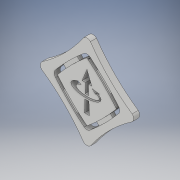
# Autodesk Inventor part: IEEE 3D
Saved by Autodesk Inventor 2018 (Build 220112000, 112)
## iProperties
Created: 2017-04-26
Part Number: IEEE 3D
Material: Generic
Document SubType Name: Modeling
Designer: Docente
Density: 1 g/cm^3
Appearance: Default
Author: Docente
Autodesk Inventor part; units mm, degrees
sketch "Sketch1" plane through (0, 0, 0) normal (0, 0, 1) x (1, 0, 0)
  line L0 (0, 0) -> (40, 0) construction
  line L1 (40, 0) -> (40, 40) construction
  line L2 (40, 40) -> (0, 40) construction
  line L3 (0, 40) -> (0, 0) construction
  line L4 (21.4142, 38.5858) -> (38.5858, 21.4142)
  line L5 (21.4142, 1.4142) -> (38.5858, 18.5858)
  line L6 (18.5858, 1.4142) -> (1.4142, 18.5858)
  line L7 (18.5858, 38.5858) -> (1.4142, 21.4142)
  arc A0 (21.4142, 38.5858) -> (18.5858, 38.5858) centre (20, 37.1716) ccw
  arc A1 (38.5858, 18.5858) -> (38.5858, 21.4142) centre (37.1716, 20) ccw
  arc A2 (18.5858, 1.4142) -> (21.4142, 1.4142) centre (20, 2.8284) ccw
  arc A3 (1.4142, 21.4142) -> (1.4142, 18.5858) centre (2.8284, 20) ccw
  line L8 (20, 0) -> (20, 20) construction
  line L9 (20, 20) -> (40, 20) construction
  line L10 (20, 20) -> (76.5685, 76.5685) construction
  line L11 (20, 20) -> (100, 20) construction
  line L12 (20, 20) -> (76.5685, -36.5685) construction
  line L13 (20, 20) -> (100, 20) construction
  line L14 (20, 20) -> (-36.5685, 76.5685) construction
  line L15 (20, 20) -> (100, 20) construction
  line L16 (20, 20) -> (-36.5685, -36.5685) construction
  line L17 (20, 20) -> (100, 20) construction
  line L18 (37.1716, 20) -> (38.5858, 21.4142) construction
  line L19 (37.1716, 20) -> (38.5858, 18.5858) construction
  line L20 (20, 37.1716) -> (21.4142, 38.5858) construction
  line L21 (20, 37.1716) -> (18.5858, 38.5858) construction
  circle A4 centre (76.5685, 76.5685) radius 66.9678
  circle A5 centre (76.5685, -36.5685) radius 66.9678
  circle A6 centre (-36.5685, -36.5685) radius 66.9678
  circle A7 centre (-36.5685, 76.5685) radius 66.9678
  point P0 (20, 40)
  point P1 (20, 0)
  point P2 (0, 20)
  dimension "d0" = 40
  dimension "d1" = 40
  dimension "d7" = 2
  dimension "d8" = 20
  dimension "d13" = 20
  dimension "d14" = 80
  dimension "d15" = 45
  dimension "d16" = 80
  dimension "d17" = 45
  dimension "d18" = 80
  dimension "d19" = 135
  dimension "d20" = 80
  dimension "d21" = 135
  constraints: 44 end point, 8 point on circle, 8 point on line, 8 tangent, 5 horizontal, 4 centre point, 4 coincident, 4 equal length, 4 midpoint, 3 equal radius, 2 parallel, 2 perpendicular, 1 vertical, 12 other
  measures "d0" distance of L2.end L1.end
  measures "d1" distance of L1.end L0.end
  measures "d7" radius of A0
  measures "d8" distance between parallel lines of L3 L8
  measures "d13" distance between parallel lines of L0 L9
  measures "d14" distance of L8.end L10.end
  measures "d15" angle of L11 L10
  measures "d16" distance of L8.end L12.end
  measures "d17" angle of L12 L13
  measures "d18" distance of L8.end L14.end
  measures "d19" angle of L15 L14
  measures "d20" distance of L8.end L16.end
  measures "d21" angle of L16 L17
extrude "Extrusion3" add sketch "Sketch1" along normal blind 2.5 contours A4 A1 A5 A2 A6 A3 A7 A0 | L4 A4 | A7 L7 | L5 A5 | A6 L6
extrude "Extrusion4" cut sketch "Sketch1" along normal blind 3.5 contours A4 A7 A5 L4 | L4 A4 | A7 L7 | L7 A7 A6 A4 | A4 A7 | A5 A4 A6 L5 | L5 A5 | A5 A4 | A6 L6 | L6 A6 A5 A7 | A7 A6 | A6 A5
ref_plane "Work Plane1" through (20, 0, 0) normal (1, 0, 0) x (0, 1, 0)
sketch "Sketch6" plane through (0, 0, 2.5) normal (0, 0, 1) x (1, 0, 0)
  line L0 (18.5858, 38.5858) -> (1.4142, 21.4142) construction
  line L1 (18.5858, 1.4142) -> (1.4142, 18.5858) construction
  line L2 (21.4142, 1.4142) -> (38.5858, 18.5858) construction
  line L3 (21.4142, 38.5858) -> (38.5858, 21.4142) construction
  arc A0 (21.4142, 38.5858) -> (18.5858, 38.5858) centre (20, 37.1716) ccw construction
  arc A1 (1.4142, 21.4142) -> (1.4142, 18.5858) centre (2.8284, 20) ccw construction
  arc A2 (18.5858, 1.4142) -> (21.4142, 1.4142) centre (20, 2.8284) ccw construction
  arc A3 (38.5858, 18.5858) -> (38.5858, 21.4142) centre (37.1716, 20) ccw construction
  line L4 (2.8284, 20) -> (20, 37.1716) construction
  line L5 (20, 37.1716) -> (37.1716, 20) construction
  line L6 (20, 2.8284) -> (37.1716, 20) construction
  line L7 (20, 2.8284) -> (2.8284, 20) construction
  line L8 (18.5858, 32.9289) -> (7.0711, 21.4142) construction
  line L9 (7.0711, 18.5858) -> (18.5858, 7.0711) construction
  line L10 (21.4142, 7.0711) -> (32.9289, 18.5858) construction
  line L11 (32.9289, 21.4142) -> (21.4142, 32.9289) construction
  arc A4 (21.4142, 32.9289) -> (18.8688, 33.1641) centre (20, 31.5147) ccw
  arc A5 (33.1641, 18.8688) -> (33.1641, 21.1312) centre (31.5147, 20) ccw
  arc A6 (18.8688, 6.8359) -> (21.4142, 7.0711) centre (20, 8.4853) ccw
  arc A7 (7.0711, 21.4142) -> (7.0711, 18.5858) centre (8.4853, 20) ccw
  line L12 (20, 31.5147) -> (20, 8.4853) construction
  line L13 (8.4853, 20) -> (31.5147, 20) construction
  line L14 (20, 20) -> (76.5685, 76.5685) construction
  line L15 (20, 20) -> (100, 20) construction
  arc A8 (7.0711, 18.5858) -> (18.8688, 6.8359) centre (76.5685, 76.5685) ccw
  line L16 (20, 20) -> (-36.5685, 76.5685) construction
  arc A9 (21.4142, 7.0711) -> (33.1641, 18.8688) centre (-36.5685, 76.5685) ccw
  line L17 (20, 20) -> (-36.5685, -36.5685) construction
  line L18 (20, 20) -> (76.5685, -36.5685) construction
  arc A10 (18.8688, 33.1641) -> (7.0711, 21.4142) centre (76.5685, -36.5685) ccw
  arc A11 (33.1641, 21.1312) -> (21.4142, 32.9289) centre (-36.5685, -36.5685) ccw
  point P0 (0, 0)
  dimension "d41" = 2
  dimension "d42" = 2
  dimension "d43" = 80
  dimension "d44" = 45
  constraints: 30 end point, 16 point on circle, 8 centre point, 8 tangent, 6 perpendicular, 4 coincident, 3 equal radius, 3 symmetric about line, 2 horizontal, 1 equal length, 1 midpoint, 1 vertical, 3 other
  measures "d41" distance between parallel lines of L4 L8
  measures "d42" radius of A4
  measures "d43" distance of L14.start L14.end
  measures "d44" angle of L15 L14
sketch "Sketch7" plane through (20, 0, 0) normal (1, 0, 0) x (0, 1, 0)
  line L0 (33.5147, 2.5) -> (32.9289, 2.5) construction
  line L1 (33.5147, 2.5) -> (32.0147, 2.5)
  line L2 (32.0147, 2.5) -> (32.0147, -1)
  line L3 (32.0147, -1) -> (33.5147, -1)
  line L4 (33.5147, -1) -> (33.5147, 2.5)
  point P0 (0, 0)
  point P1 (33.1641, 2.5)
  dimension "d45" = 1.5
  dimension "d46" = 3.5
  constraints: 8 end point, 2 parallel, 1 horizontal, 1 perpendicular
  measures "d45" distance of L3.end L2.end
  measures "d46" distance of L2.end L1.end
sweep "Sweep1" cut profiles "Sketch7" path "Sketch6"
sketch "Sketch8" plane through (0, 0, 2.5) normal (0, 0, 1) x (1, 0, 0)
  line L0 (20, 20) -> (-36.5685, 76.5685) construction
  line L1 (20, 20) -> (76.5685, -36.5685) construction
  line L2 (20, 20) -> (-36.5685, -36.5685) construction
  line L3 (20, 20) -> (76.5685, 76.5685) construction
  line L4 (20, 20) -> (11.3989, 28.6011)
  line L5 (20, 31.5147) -> (20, 8.4853) construction
  line L6 (20, 20) -> (76.5685, 76.5685) construction
  point P0 (0, 0)
  constraints: 4 end point, 1 point on line
ref_plane "Work Plane2" through (11.3989, 28.6011, 2.5) normal (-0.7071, 0.7071, 0) x (-0.7071, -0.7071, 0)
sketch "Sketch9" plane through (11.3989, 28.6011, 2.5) normal (-0.7071, 0.7071, 0) x (-0.7071, -0.7071, 0)
  line L0 (0, -0.5) -> (0, 0)
  line L1 (-4, -2) -> (4, -2)
  line L2 (4, -2) -> (4, -0.5)
  line L3 (4, -0.5) -> (-4, -0.5)
  line L4 (-4, -0.5) -> (-4, -2)
  point P0 (28.2843, -2.5)
  dimension "d52" = 0.5
  dimension "d53" = 8
  dimension "d54" = 1.5
  constraints: 10 end point, 2 parallel, 1 coincident, 1 horizontal, 1 midpoint, 1 perpendicular, 1 vertical
  measures "d52" distance of L0.start L0.end
  measures "d53" distance of L3.end L2.end
  measures "d54" distance of L2.end L1.end
sweep "Sweep2" add profiles "Sketch9" path "Sketch8"
mirror "Mirror1" about plane through (20, 0, 0) normal (1, 0, 0) of "Sweep2"
ref_plane "Work Plane3" through (0, 20, 0) normal (0, 1, 0) x (-1, 0, 0)
mirror "Mirror2" about plane through (0, 20, 0) normal (0, 1, 0) of "Sweep2", "Mirror1"
sketch "Sketch10" plane through (20, 0, 0) normal (1, 0, 0) x (0, 1, 0)
  point P0 (0, 0)
sketch "Sketch11" plane through (0, 0, 2.5) normal (0, 0, 1) x (1, 0, 0)
  line L0 (20, 28) -> (20, 12) construction
  line L1 (19, 12) -> (21, 12)
  line L2 (19.5, 25) -> (20.5, 25) construction
  line L3 (20, 28) -> (20, 25) construction
  line L4 (21, 12) -> (20.5, 25)
  line L5 (19, 12) -> (19.5, 25)
  line L6 (20, 28) -> (25.5169, 28) construction
  line L7 (20, 28) -> (20, 23) construction
  line L8 (20, 23) -> (18, 23)
  line L9 (18, 23) -> (20, 28)
  line L10 (20, 23) -> (22, 23)
  line L11 (22, 23) -> (20, 28)
  line L12 (19.4231, 23) -> (20.5769, 23)
  line L13 (20, 20) -> (20, 18.7353) construction
  arc A0 (19.2704, 19.0296) -> (20.7296, 19.0296) centre (20, 28) ccw
  arc A1 (19.1934, 17.0296) -> (20.8066, 17.0296) centre (20, 28) ccw
  line L14 (19.2704, 19.0296) -> (19.4231, 23)
  line L15 (19.4231, 23) -> (20.5769, 23)
  line L16 (20.5769, 23) -> (20.7296, 19.0296)
  line L17 (19, 12) -> (19.1934, 17.0296)
  line L18 (20.8066, 17.0296) -> (21, 12)
  line L19 (19, 12) -> (21, 12)
  line L20 (21, 12) -> (20.8066, 17.0296)
  point P0 (0, 0)
  dimension "d58" = 16
  dimension "d59" = 2
  dimension "d60" = 1
  dimension "d61" = 3
  dimension "d65" = 5
  dimension "d66" = 2
  dimension "d88" = 9
  dimension "d89" = 11
  constraints: 42 end point, 9 point on line, 7 collinear, 4 horizontal, 4 point on circle, 3 coincident, 3 midpoint, 2 centre point, 1 symmetric about line, 1 vertical
  measures "d58" distance of L0.end L0.start
  measures "d59" distance of L1.start L1.end
  measures "d60" distance of L2.start L2.end
  measures "d61" distance of L3.end L0.start
  measures "d65" distance of L0.start L7.end
  measures "d66" distance of L7.end L8.end
  measures "d88" radius of A0
  measures "d89" radius of A1
sketch "Sketch12" plane through (0, 0, 2.5) normal (0, 0, 1) x (1, 0, 0)
  line L0 (21, 12) -> (20.5, 25) construction
  ellipse E0 centre (20.3, 20) end of major axis (25.0589, 20) minor radius 1.6476 (17.6355, 21.3651) -> (21.5863, 21.5863) ccw
  ellipse E1 centre (19.6, 20) end of major axis (13.4024, 20) minor radius 2.3878 (16.4416, 22.0545) -> (22.1724, 22.1724) ccw
  line L1 (20, 20) -> (20.3, 20) construction
  line L2 (20, 20) -> (19.6, 20) construction
  line L3 (20, 20) -> (16.4718, 22.037) construction
  line L4 (20, 20) -> (24.074, 20) construction
  line L5 (17.6355, 21.3651) -> (16.4416, 22.0545) construction
  line L6 (22.1724, 22.1724) -> (25.1343, 21.6955)
  line L7 (19.9483, 19.9104) -> (22.2046, 22.1667) construction
  line L8 (19.9483, 19.9104) -> (23.1392, 19.9104) construction
  line L9 (20, 20) -> (22.465, 22.465) construction
  line L10 (20, 20) -> (23.486, 20) construction
  line L11 (22.1724, 22.1724) -> (23.4452, 20.8996)
  line L12 (22.1724, 22.1724) -> (23.9724, 22.1724) construction
  line L13 (23.4452, 20.8996) -> (25.1343, 21.6955)
  line L14 (16.4416, 22.0545) -> (17.6355, 21.3651)
  line L15 (23.858, 21.0941) -> (24.5669, 21.4281)
  point P0 (0, 0)
  dimension "d72" = 6.1976
  dimension "d73" = 2.3878
  dimension "d74" = 4.7589
  dimension "d75" = 1.6476
  dimension "d70" = 0.3
  dimension "d71" = 0.4
  dimension "d76" = 150
  dimension "d77" = 3
  dimension "d78" = 45
  dimension "d79" = 45
  dimension "d80" = 2.9619
  dimension "d81" = 1.8
  dimension "d82" = 45
  constraints: 30 end point, 6 horizontal, 6 point on line, 4 equal length, 2 coincident, 1 collinear, 11 other
  measures "d70" distance of L1.start L1.end
  measures "d71" distance of L1.start L2.end
  measures "d76" angle of L4 L3
  measures "d77" distance of L6.start L6.end
  measures "d78" angle of L8 L7
  measures "d79" angle of L10 L9
  measures "d80" horizontal distance of L6.start L6.end
  measures "d81" distance of L6.start L11.end
  measures "d82" angle of L11 L12
extrude "Extrusion7" cut sketch "Sketch11" against normal blind 4 contours L5 A1 L4 L1 | L5 L8 L10 L4 A0 | L8 L9 L11 L10
extrude "Extrusion8" cut sketch "Sketch12" against normal blind 4
body "Solid3"
